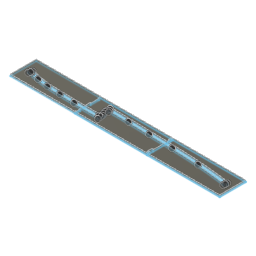
_single scale fb.bcdadba6-970f-41f2-bbc7-cf30ff8ed793 (Autodesk Fusion 360 design; units mm, degrees)
Autodesk Fusion 360 part; units mm, degrees
sketch "Sketch1" plane through (0, 0, 0) normal (0, 0, 1) x (1, 0, 0)
  line L0 (0, 0) -> (0, 38.1)
  line L1 (0, 19.05) -> (-648.75, 19.05)
  line L2 (-648.75, -9.7125) -> (-648.75, 47.8125)
  line L3 (0, 0) -> (-648.75, -9.7125)
  line L4 (0, 38.1) -> (-648.75, 47.8125)
  line L5 (0, 38.1) -> (0, 35.1)
  line L6 (0, 0) -> (-0.0032, 0.2146)
  line L7 (0, 0) -> (0, 3)
  line L8 (0, 19.05) -> (-865, 19.05)
  line L9 (-865, 48.05) -> (-865, -9.95)
  line L10 (-865, 48.05) -> (0, 35.1)
  line L11 (0, 3) -> (-865, -9.95)
  line L12 (-635.8911, 47.62) -> (-635.8911, -9.52)
  line L13 (-622.2676, 47.416) -> (-622.2676, -9.316)
  line L14 (-607.834, 47.1999) -> (-607.834, -9.0999)
  line L15 (-592.5421, 46.971) -> (-592.5421, -8.871)
  line L16 (-576.3409, 46.7285) -> (-576.3409, -8.6285)
  line L17 (-559.1763, 46.4715) -> (-559.1763, -8.3715)
  line L18 (-540.9911, 46.1992) -> (-540.9911, -8.0992)
  line L19 (-479.6863, 45.2814) -> (-479.6863, -7.1814)
  line L20 (-521.7245, 45.9108) -> (-521.7245, -7.8108)
  line L21 (-501.3123, 45.6052) -> (-501.3123, -7.5052)
  line L22 (-456.7744, 44.9384) -> (-456.7744, -6.8384)
  line L23 (-432.5, 44.575) -> (-432.5, -6.475)
  line L24 (-406.7822, 44.19) -> (-406.7822, -6.09)
  line L25 (-379.5352, 43.7821) -> (-379.5352, -5.6821)
  line L26 (-350.6679, 43.3499) -> (-350.6679, -5.2499)
  line L27 (-320.0841, 42.892) -> (-320.0841, -4.792)
  line L28 (-287.6818, 42.4069) -> (-287.6818, -4.3069)
  line L29 (-253.3526, 41.893) -> (-253.3526, -3.793)
  line L30 (-216.9822, 41.3485) -> (-216.9822, -3.2485)
  line L31 (-178.449, 40.7716) -> (-178.449, -2.6716)
  line L32 (-137.6246, 40.1604) -> (-137.6246, -2.0604)
  line L33 (-94.3726, 39.5129) -> (-94.3726, -1.4129)
  line L34 (-48.5491, 38.7707) -> (-48.5491, -0.7268)
  dimension "d30" = 38.1
  dimension "d31" = 3
  dimension "d32" = 3
  dimension "d33" = 865
  dimension "d34" = 58
  dimension "d35" = 648.75
  dimension "d36" = 635.8911
  dimension "d37" = 622.2676
  dimension "d38" = 607.834
  dimension "d39" = 592.5421
  dimension "d40" = 576.3409
  dimension "d41" = 559.1763
  dimension "d42" = 540.9911
  dimension "d43" = 521.7245
  dimension "d44" = 501.3123
  dimension "d45" = 479.6863
  dimension "d46" = 456.7744
  dimension "d47" = 432.5
  dimension "d48" = 48.5491
  dimension "d49" = 94.3726
  dimension "d50" = 137.6246
  dimension "d51" = 178.449
  dimension "d52" = 216.9822
  dimension "d53" = 253.3526
  dimension "d54" = 287.6818
  dimension "d55" = 320.0841
  dimension "d56" = 350.6679
  dimension "d57" = 379.5352
  dimension "d58" = 406.7822
  constraint coincident L0.start L3.start
  constraint vertical L0
  constraint midpoint L0 L1.start
  constraint perpendicular L0 L1
  constraint vertical L2
  constraint midpoint L1.end L2
  constraint coincident L0 L5.end
  constraint parallel L0 L5
  constraint perpendicular L3 L6
  constraint coincident L0 L7.end
  constraint perpendicular L0 L8
  constraint vertical L9
  constraint midpoint L8.end L9
  constraint parallel L4 L10
  constraint coincident L4 L12.start
  constraint coincident L3 L12.end
  constraint coincident L4 L13.start
  constraint coincident L3 L13.end
  constraint coincident L4 L14.start
  constraint coincident L3 L14.end
  constraint perpendicular L8 L12
  constraint perpendicular L1 L13
  constraint perpendicular L8 L14
  constraint coincident L4 L15.start
  constraint coincident L3 L15.end
  constraint coincident L3 L16.end
  constraint coincident L4 L17.start
  constraint coincident L3 L17.end
  constraint coincident L4 L16.start
  constraint coincident L4 L18.start
  constraint coincident L3 L18.end
  constraint coincident L4 L19.start
  constraint coincident L3 L19.end
  constraint coincident L4 L20.start
  constraint coincident L3 L20.end
  constraint parallel L19 L20
  constraint coincident L4 L21.start
  constraint coincident L3 L21.end
  constraint parallel L20 L21
  constraint coincident L4 L22.start
  constraint coincident L3 L22.end
  constraint coincident L4 L23.start
  constraint coincident L3 L23.end
  constraint perpendicular L1 L15
  constraint perpendicular L1 L16
  constraint perpendicular L8 L17
  constraint perpendicular L8 L18
  constraint perpendicular L1 L19
  constraint perpendicular L1 L22
  constraint perpendicular L1 L23
  constraint coincident L4 L24.start
  constraint coincident L3 L24.end
  constraint coincident L4 L25.start
  constraint coincident L3 L25.end
  constraint coincident L4 L26.start
  constraint coincident L3 L26.end
  constraint coincident L4 L27.start
  constraint coincident L3 L27.end
  constraint coincident L4 L28.start
  constraint coincident L3 L28.end
  constraint coincident L4 L29.start
  constraint coincident L3 L29.end
  constraint coincident L4 L30.start
  constraint coincident L3 L30.end
  constraint coincident L4 L31.start
  constraint coincident L3 L31.end
  constraint coincident L4 L32.start
  constraint coincident L3 L32.end
  constraint coincident L4 L33.start
  constraint coincident L3 L33.end
  constraint coincident L3 L34.end
  constraint parallel L32 L34
  constraint perpendicular L8 L24
  constraint perpendicular L1 L25
  constraint perpendicular L8 L26
  constraint perpendicular L8 L27
  constraint perpendicular L1 L28
  constraint perpendicular L8 L29
  constraint perpendicular L1 L30
  constraint perpendicular L1 L31
  constraint perpendicular L8 L32
  constraint perpendicular L8 L33
  measures "d30" distance of L0.start L0.end
  measures "d31" distance of L0.end L5.end
  measures "d32" distance of L0.start L7.end
  measures "d33" distance of L1.start L8.end
  measures "d34" distance of L9.start L9.end
  measures "d35" distance of L0 L2
  measures "d36" distance of L0 L12
  measures "d37" distance of L0 L13
  measures "d38" distance of L0 L14
  measures "d39" distance of L0 L15
  measures "d40" distance of L0 L16
  measures "d41" distance of L0 L17
  measures "d42" distance of L0 L18
  measures "d43" distance of L0 L20
  measures "d44" distance of L0 L21
  measures "d45" distance of L0 L19
  measures "d46" distance of L0 L22
  measures "d47" distance of L0 L23
  measures "d48" distance of L0 L34
  measures "d49" distance of L0 L33
  measures "d50" distance of L0 L32
  measures "d51" distance of L0 L31
  measures "d52" distance of L0 L30
  measures "d53" distance of L0 L29
  measures "d54" distance of L0 L28
  measures "d55" distance of L0 L27
  measures "d56" distance of L0 L26
  measures "d57" distance of L0 L25
  measures "d58" distance of L0 L24
extrude "Extrude1" add sketch "Sketch1" along normal blind 1 contours L3 L11 L33 L34 | L1 L8 L11 L33 L34 | L0 L4 L5 L10 L33 | L1 L8 L10 L33 L34 | L3 L11 L31 L32 | L1 L8 L11 L31 L32 | L1 L8 L10 L31 L32 | L3 L11 L29 L30 | L4 L10 L31 L32 | L1 L8 L11 L29 L30 | L1 L8 L10 L29 L30 | L3 L11 L27 L28 | L4 L10 L29 L30 | L1 L8 L11 L27 L28 | L1 L8 L10 L27 L28 | L3 L11 L25 L26 | L4 L10 L27 L28 | L1 L8 L11 L25 L26 | L1 L8 L10 L25 L26 | L3 L11 L23 L24 | L4 L10 L25 L26 | L1 L8 L11 L23 L24 | L1 L8 L10 L23 L24 | L3 L11 L19 L22 | L4 L10 L23 L24 | L1 L8 L11 L19 L22 | L1 L8 L10 L19 L22 | L3 L11 L20 L21 | L4 L10 L19 L22 | L1 L8 L11 L20 L21 | L1 L8 L10 L20 L21 | L3 L11 L17 L18 | L4 L10 L20 L21 | L1 L8 L11 L17 L18 | L1 L8 L10 L17 L18 | L3 L11 L15 L16 | L4 L10 L17 L18 | L1 L8 L11 L15 L16 | L1 L8 L10 L15 L16 | L3 L11 L13 L14 | L4 L10 L15 L16 | L1 L8 L11 L13 L14 | L1 L8 L10 L13 L14 | L2 L3 L11 L12 | L4 L10 L13 L14 | L1 L2 L8 L11 L12 | L1 L2 L8 L10 L12 | L2 L4 L10 L12 makes body 1 at (-79.0981, 24.6423, 0) makes body 2 at (-472.049, 10.4205, 0) makes body 3 at (-617.4564, 9.6667, 0) makes body 4 at (-587.1417, 9.8238, 0) makes body 5 at (-423.9274, 10.67, 0) makes body 6 at (-241.2292, 11.6172, 0) makes body 7 at (-164.8409, 12.0132, 0) makes body 8 at (-514.9204, 10.1983, 0) makes body 9 at (-644.4637, 9.5267, 0) makes body 10 at (-553.1146, 10.0003, 0) makes body 11 at (-309.2834, 11.2644, 0) makes body 12 at (-369.9128, 10.95, 0)
extrude "Extrude2" add sketch "Sketch1" along normal blind 1.1 contours L0 L3 L7 L11 L34 | L0 L1 L8 L11 L34 | L0 L1 L8 L10 L34 | L3 L11 L32 L33 | L0 L4 L5 L10 L33 | L1 L8 L11 L32 L33 | L1 L8 L10 L32 L33 | L3 L11 L30 L31 | L4 L10 L32 L33 | L1 L8 L11 L30 L31 | L1 L8 L10 L30 L31 | L3 L11 L28 L29 | L4 L10 L30 L31 | L1 L8 L11 L28 L29 | L1 L8 L10 L28 L29 | L3 L11 L26 L27 | L4 L10 L28 L29 | L1 L8 L11 L26 L27 | L1 L8 L10 L26 L27 | L3 L11 L24 L25 | L4 L10 L26 L27 | L1 L8 L11 L24 L25 | L1 L8 L10 L24 L25 | L3 L11 L22 L23 | L4 L10 L24 L25 | L1 L8 L11 L22 L23 | L1 L8 L10 L22 L23 | L3 L11 L19 L21 | L4 L10 L22 L23 | L1 L8 L11 L19 L21 | L1 L8 L10 L19 L21 | L3 L11 L18 L20 | L4 L10 L19 L21 | L1 L8 L11 L18 L20 | L1 L8 L10 L18 L20 | L3 L11 L16 L17 | L4 L10 L18 L20 | L1 L8 L11 L16 L17 | L1 L8 L10 L16 L17 | L3 L11 L14 L15 | L4 L10 L16 L17 | L1 L8 L11 L14 L15 | L1 L8 L10 L14 L15 | L3 L11 L12 L13 | L4 L10 L14 L15 | L1 L8 L11 L12 L13 | L1 L8 L10 L12 L13 | L4 L10 L12 L13 bodies 1 2 3 4 5 6 7 8 9 10 11 12
sketch "Sketch2" plane through (0, 0, 0) normal (0, 0, 1) x (1, 0, 0)
  spline S0 degree 5 poles (-24.1605, 18.6518) (-27.5504, 19.122) (-34.3155, 20.0408) (-44.4187, 21.3547) (-57.8005, 22.9772) (-74.3771, 24.7888) (-90.7994, 26.384) (-107.0622, 27.7655) (-123.1579, 28.9406) (-139.077, 29.9226) (-154.8084, 30.7321) (-170.3409, 31.3938) (-185.6653, 31.9351) (-200.7758, 32.384) (-215.6719, 32.7674) (-230.3606, 33.1094) (-244.8532, 33.4302) (-259.1638, 33.745) (-273.3065, 34.0635) (-287.2938, 34.3883) (-301.1346, 34.7142) (-314.835, 35.0314) (-328.3992, 35.3278) (-341.8301, 35.5915) (-355.1302, 35.8137) (-368.3019, 35.9899) (-378.7381, 36.0923) (-386.509, 36.1472) (-391.6646, 36.1741) (-394.2362, 36.1852) knots 0 0 0 0 0 0 0.04 0.08 0.12 0.16 0.2 0.24 0.28 0.32 0.36 0.4 0.44 0.48 0.52 0.56 0.6 0.64 0.68 0.72 0.76 0.8 0.84 0.88 0.92 0.96 1 1 1 1 1 1
  spline S1 degree 5 poles (-392.9597, 2.1867) (-395.6742, 2.1899) (-401.039, 2.1986) (-408.893, 2.2191) (-418.9781, 2.2614) (-430.9371, 2.3391) (-442.252, 2.4411) (-452.9376, 2.5661) (-463.0261, 2.7117) (-472.5725, 2.8738) (-481.6645, 3.0465) (-490.4181, 3.2224) (-498.9558, 3.3967) (-507.3876, 3.5702) (-515.7938, 3.7524) (-524.2015, 3.9653) (-532.5808, 4.2437) (-540.8725, 4.627) (-549.0091, 5.1533) (-556.936, 5.8532) (-564.6381, 6.7419) (-572.1386, 7.8197) (-579.4807, 9.0786) (-586.7153, 10.5058) (-593.8853, 12.0894) (-601.0154, 13.8215) (-606.6978, 15.3222) (-610.9493, 16.5114) (-613.7791, 17.3323) (-615.1929, 17.7498) knots 0 0 0 0 0 0 0.04 0.08 0.12 0.16 0.2 0.24 0.28 0.32 0.36 0.4 0.44 0.48 0.52 0.56 0.6 0.64 0.68 0.72 0.76 0.8 0.84 0.88 0.92 0.96 1 1 1 1 1 1
  spline S2 degree 5 poles (-394.2362, 36.1852) (-394.4192, 35.9036) (-394.7704, 35.3375) (-395.2523, 34.4799) (-395.8052, 33.3193) (-396.3447, 31.8405) (-396.7298, 30.3356) (-396.9561, 28.8089) (-397.0185, 27.2679) (-396.9105, 25.7246) (-396.6265, 24.194) (-396.1673, 22.6915) (-395.5434, 21.23) (-394.7797, 19.8172) (-393.9211, 18.4527) (-393.0333, 17.1263) (-392.1909, 15.8233) (-391.4662, 14.5276) (-390.9189, 13.2259) (-390.5844, 11.9118) (-390.463, 10.5898) (-390.5297, 9.2715) (-390.7459, 7.9726) (-391.0695, 6.7087) (-391.4668, 5.4919) (-391.9183, 4.3287) (-392.3147, 3.4433) (-392.6302, 2.8051) (-392.8485, 2.3909) (-392.9597, 2.1867) knots 0 0 0 0 0 0 0.04 0.08 0.12 0.16 0.2 0.24 0.28 0.32 0.36 0.4 0.44 0.48 0.52 0.56 0.6 0.64 0.68 0.72 0.76 0.8 0.84 0.88 0.92 0.96 1 1 1 1 1 1
  spline S3 degree 3 poles (-23.3972, 24.1554) (-53.7424, 28.3641) (-83.4113, 31.5287) (-112.2795, 33.6915) (-140.6174, 35.8146) (-168.1418, 36.9676) (-194.6063, 37.7506) (-218.9869, 38.4719) (-242.4676, 38.9277) (-265.2955, 39.4418) (-290.8491, 40.0174) (-315.6411, 40.6541) (-339.8372, 41.1024) (-358.3233, 41.445) (-376.4448, 41.6651) (-394.2123, 41.7413) (-395.2225, 41.7457) (-396.2327, 41.75) (-397.2429, 41.7544) knots 0 0 0 0 0.214055 0.214055 0.214055 0.424177 0.424177 0.424177 0.617755 0.617755 0.617755 0.834445 0.834445 0.834445 1 1 1 1.009428 1.009428 1.009428 1.009428
  spline S4 degree 3 poles (-397.2429, 41.7544) (-397.7935, 40.9074) (-398.3441, 40.0604) (-398.8947, 39.2134) (-400.9484, 36.0541) (-402.2505, 32.4986) (-402.4927, 28.7482) (-402.6465, 26.3683) (-402.3521, 23.8989) (-401.6161, 21.5883) (-400.8898, 19.3082) (-399.7176, 17.2208) (-398.6655, 15.5787) (-397.7882, 14.2096) (-397.0465, 13.1262) (-396.6414, 12.3604) (-396.2385, 11.5989) (-396.1333, 11.2077) (-396.0845, 10.7672) (-396.0384, 10.3511) (-396.0661, 9.82) (-396.21, 9.1253) (-396.2986, 8.6979) (-396.4291, 8.2227) (-396.5851, 7.7481) knots -0.072189 -0.072189 -0.072189 -0.072189 0 0 0 0.210827 0.210827 0.210827 0.344606 0.344606 0.344606 0.476616 0.476616 0.476616 0.586683 0.586683 0.586683 0.696118 0.696118 0.696118 0.799473 0.799473 0.799473 0.863067 0.863067 0.863067 0.863067
  spline S5 degree 3 poles (-396.5851, 7.7481) (-412.9972, 7.7754) (-427.9476, 7.8595) (-441.4582, 7.9968) (-453.4386, 8.1186) (-464.2646, 8.2834) (-474.2943, 8.4668) (-484.668, 8.6565) (-494.2501, 8.8557) (-503.7387, 9.0534) (-511.748, 9.2202) (-519.7124, 9.3836) (-527.6043, 9.6481) (-536.5484, 9.948) (-545.3312, 10.3976) (-553.6662, 11.1703) (-566.0615, 12.3194) (-577.488, 14.1948) (-588.7791, 16.6726) (-597.1203, 18.503) (-605.3869, 20.6474) (-613.6191, 23.0786) knots 0.01078 0.01078 0.01078 0.01078 0.157894 0.157894 0.157894 0.288347 0.288347 0.288347 0.423272 0.423272 0.423272 0.537163 0.537163 0.537163 0.666241 0.666241 0.666241 0.858196 0.858196 0.858196 1 1 1 1
  spline S6 degree 3 poles (-24.925, 13.1396) (-56.1966, 17.4768) (-86.7138, 20.6902) (-116.3791, 22.8424) (-146.2599, 25.0102) (-175.2477, 26.1059) (-203.1333, 26.867) (-227.0891, 27.5209) (-250.2459, 27.9729) (-272.8003, 28.4879) (-305.7283, 29.2398) (-337.3904, 30.0519) (-368.0168, 30.4095) (-375.6935, 30.4992) (-383.3047, 30.564) (-390.8514, 30.6039) knots 0 0 0 0 0.222207 0.222207 0.222207 0.44603 0.44603 0.44603 0.63831 0.63831 0.63831 0.919028 0.919028 0.919028 0.989393 0.989393 0.989393 0.989393
  spline S7 degree 3 poles (-390.8514, 30.6039) (-391.2771, 29.4114) (-391.4534, 28.2523) (-391.4049, 27.1205) (-391.3499, 25.839) (-391.0275, 24.6525) (-390.2822, 23.2346) (-389.7416, 22.2059) (-388.9237, 21.0302) (-387.9756, 19.5405) (-387.1981, 18.3189) (-386.3443, 16.8569) (-385.7518, 15.1566) (-385.195, 13.5589) (-384.9244, 11.7976) (-384.9436, 10.192) (-384.9662, 8.2966) (-385.3201, 6.6335) (-385.7431, 5.1708) (-386.3578, 3.0455) (-387.1404, 1.2368) (-388.0724, -0.4747) (-388.6001, -1.4438) (-389.1279, -2.4129) (-389.6556, -3.3821) knots 0.102754 0.102754 0.102754 0.102754 0.25 0.25 0.25 0.416722 0.416722 0.416722 0.537678 0.537678 0.537678 0.636869 0.636869 0.636869 0.73008 0.73008 0.73008 0.840112 0.840112 0.840112 1 1 1 1.113902 1.113902 1.113902 1.113902
  spline S8 degree 3 poles (-389.6556, -3.3821) (-390.7591, -3.3808) (-391.8626, -3.3795) (-392.9661, -3.3783) (-411.1084, -3.3574) (-427.5197, -3.2689) (-442.2288, -3.1171) (-454.1895, -2.9936) (-465.0039, -2.8271) (-475.0197, -2.643) (-485.8695, -2.4435) (-495.8413, -2.2365) (-505.7683, -2.0278) (-513.8314, -1.8583) (-521.8904, -1.6885) (-529.936, -1.3988) (-539.2101, -1.0649) (-548.3977, -0.5483) (-557.1746, 0.3366) (-572.2612, 1.8578) (-586.1154, 4.4555) (-599.8191, 7.8248) (-605.4971, 9.2208) (-611.143, 10.7512) (-616.7691, 12.4127) knots -0.009757 -0.009757 -0.009757 -0.009757 0 0 0 0.160278 0.160278 0.160278 0.290608 0.290608 0.290608 0.431792 0.431792 0.431792 0.546467 0.546467 0.546467 0.678651 0.678651 0.678651 0.905858 0.905858 0.905858 1 1 1 1
  circle A0 centre (-615.1929, 17.7498) radius 5.5563
  circle A1 centre (-24.1605, 18.6518) radius 5.5563
  line L0 (-635.387, 55.5878) -> (0.3019, 55.5878)
  line L1 (0.3019, 55.5878) -> (0.3019, -22.6366)
  line L2 (0.3019, -22.6366) -> (-635.387, -22.6366)
  line L3 (-635.387, -22.6366) -> (-635.387, 55.5878)
  line L4 (0.3019, 55.5878) -> (-219.6981, 55.5878)
  line L5 (-219.6981, 55.5878) -> (-219.6981, -22.6366)
  line L6 (-219.6981, -22.6366) -> (0.3019, -22.6366)
  line L7 (0.3019, -22.6366) -> (0.3019, 55.5878)
  line L8 (-219.6981, -22.6366) -> (-439.6981, -22.6366)
  line L9 (-439.6981, -22.6366) -> (-439.6981, 55.5878)
  line L10 (-439.6981, 55.5878) -> (-219.6981, 55.5878)
  line L11 (-219.6981, 55.5878) -> (-219.6981, -22.6366)
  line L12 (-439.6981, 46.5574) -> (-436.8266, 48.7159)
  line L13 (-436.8266, 48.7159) -> (-436.8266, 22.3408)
  line L14 (-436.8266, 22.3408) -> (-439.6981, 24.9301)
  line L15 (-439.6981, -10.813) -> (-436.9315, -9.2445)
  line L16 (-436.9315, -9.2445) -> (-436.9315, -19.86)
  line L17 (-436.9315, -19.86) -> (-439.6981, -18.5335)
  line L18 (-219.6981, -14.6793) -> (-224.7101, -18.5577)
  line L19 (-224.7101, -18.5577) -> (-224.7101, -2.3535)
  line L20 (-224.7101, -2.3535) -> (-219.6981, -4.7563)
  line L21 (-219.6981, 47.3385) -> (-223.4841, 44.4088)
  line L22 (-223.4841, 44.4088) -> (-223.4841, 52.6422)
  line L23 (-223.4841, 52.6422) -> (-219.6981, 50.8271)
  line L24 (-616.7691, 12.4127) -> (-617.5556, 12.721)
  line L25 (-24.925, 13.1396) -> (-24.3151, 13.0977)
  point P0 (-117.246, 28.4843)
  point P1 (-199.5489, 32.3347)
  point P2 (-271.2631, 34.0193)
  point P3 (-335.5171, 35.4632)
  point P4 (-468.4361, 2.8063)
  point P5 (-512.4703, 3.6834)
  point P6 (-551.9344, 5.4378)
  point P7 (-584.9597, 10.1867)
  point P8 (-396.9597, 28.1867)
  point P9 (-394.9597, 20.1867)
  point P10 (-390.9597, 13.1867)
  point P11 (-390.9597, 7.1867)
  dimension "d63" = 5.5562
  dimension "d64" = -5.565
  dimension "d65" = 220
  dimension "d66" = 220
  constraint coincident S1.end A0.centre
  constraint coincident S5.end A0
  constraint coincident S0.start A1.centre
  constraint coincident S3.start A1
  constraint horizontal L0
  constraint vertical L1
  constraint horizontal L2
  constraint vertical L3
  constraint horizontal L4
  constraint vertical L5
  constraint horizontal L6
  constraint vertical L7
  constraint coincident L2 L5.end
  constraint horizontal L8
  constraint vertical L9
  constraint horizontal L10
  constraint vertical L11
  constraint coincident L0 L9.end
  constraint coincident L9 L12.start
  constraint parallel L9 L13
  constraint coincident L9 L14.end
  constraint coincident L9 L15.start
  constraint parallel L9 L16
  constraint coincident L9 L17.end
  constraint coincident L5 L18.start
  constraint parallel L5 L19
  constraint coincident L11 L20.end
  constraint parallel L17 L20
  constraint coincident L11 L21.start
  constraint parallel L18 L21
  constraint parallel L11 L22
  constraint coincident L11 L23.end
  constraint parallel L20 L23
  constraint coincident A0 L24.end
  constraint coincident A1 L25.end
  measures "d65" distance of L0.end L4.end
  measures "d66" distance of L5.end L8.end
extrude "Extrude3" add sketch "Sketch2" along normal blind 5 separate body contours S5 S8 A0 L0 L2 L3 L9 L24 | L9 L15 L16 L17 | L9 L12 L13 L14 makes body 13
extrude "Extrude1'" add sketch "Sketch2" along normal blind 5 separate body contours S3 S4 S5 L0 L5 L9 L10 L11 L12 L13 L14 L21 L22 L23 | S6 S7 S8 L2 L5 L8 L9 L11 L15 L16 L17 L18 L19 L20 makes body 14 at (-276.582, 12.8884, 0) makes body 15 at (-425.3289, 33.7801, 0) in component "Component"
extrude "Extrude1''" add sketch "Sketch2" along normal blind 5 separate body contours S3 S6 A1 L0 L1 L2 L4 L5 L6 L7 L11 L25 | L5 L11 L21 L22 L23 | L5 L11 L18 L19 L20 makes body 16 in component "Component'"
component "Component" placed x (1, 0, 0) y (0, 1, 0) z (0, 0, 1) at (0, 0, 0)
component "Component'" placed x (1, 0, 0) y (0, 1, 0) z (0, 0, 1) at (0, 0, 0)
hidden bodies 1
equation "div = 17.817"
equation "scale = 865 mm"
equation "f1 = scale / div"
equation "f2 = scale - ( scale / 2 ^ ( 2 / 12 ) )"
equation "f3 = scale - ( scale / 2 ^ ( 3 / 12 ) )"
equation "f4 = scale - ( scale / 2 ^ ( 4 / 12 ) )"
equation "f5 = scale - ( scale / 2 ^ ( 5 / 12 ) )"
equation "f6 = scale - ( scale / 2 ^ ( 6 / 12 ) )"
equation "f7 = scale - ( scale / 2 ^ ( 7 / 12 ) )"
equation "f8 = scale - ( scale / 2 ^ ( 8 / 12 ) )"
equation "f9 = scale - ( scale / 2 ^ ( 9 / 12 ) )"
equation "f10 = scale - ( scale / 2 ^ ( 10 / 12 ) )"
equation "f11 = scale - ( scale / 2 ^ ( 11 / 12 ) )"
equation "f12 = scale - ( scale / 2 ^ ( 12 / 12 ) )"
equation "f13 = scale - ( scale / 2 ^ ( 13 / 12 ) )"
equation "f14 = scale - ( scale / 2 ^ ( 14 / 12 ) )"
equation "f15 = scale - ( scale / 2 ^ ( 15 / 12 ) )"
equation "f16 = scale - ( scale / 2 ^ ( 16 / 12 ) )"
equation "f17 = scale - ( scale / 2 ^ ( 17 / 12 ) )"
equation "f18 = scale - ( scale / 2 ^ ( 18 / 12 ) )"
equation "f19 = scale - ( scale / 2 ^ ( 19 / 12 ) )"
equation "f20 = scale - ( scale / 2 ^ ( 20 / 12 ) )"
equation "f22 = scale - ( scale / 2 ^ ( 22 / 12 ) )"
equation "f21 = scale - ( scale / 2 ^ ( 21 / 12 ) )"
equation "f23 = scale - ( scale / 2 ^ ( 23 / 12 ) )"
equation "f24 = scale - ( scale / 2 ^ ( 24 / 12 ) )"
equation "nut = 1.5 in"
equation "bridge = 58 mm"
equation "edge = 3 mm"
equation "d30 = nut"
equation "d31 = edge"
equation "d32 = edge"
equation "d33 = scale"
equation "d34 = bridge"
equation "d35 = f24"
equation "d36 = f23"
equation "d37 = f22"
equation "d38 = f21"
equation "d39 = f20"
equation "d40 = f19"
equation "d41 = f18"
equation "d42 = f17"
equation "d43 = f16"
equation "d44 = f15"
equation "d45 = f14"
equation "d46 = f13"
equation "d47 = f12"
equation "d48 = f1"
equation "d49 = f2"
equation "d50 = f3"
equation "d51 = f4"
equation "d52 = f5"
equation "d53 = f6"
equation "d54 = f7"
equation "d55 = f8"
equation "d56 = f9"
equation "d57 = f10"
equation "d58 = f11"
equation "d63 = ( 7 / 32 * 25.4 ) * 1 mm"
equation "d64 = -11.13 mm / 2"
